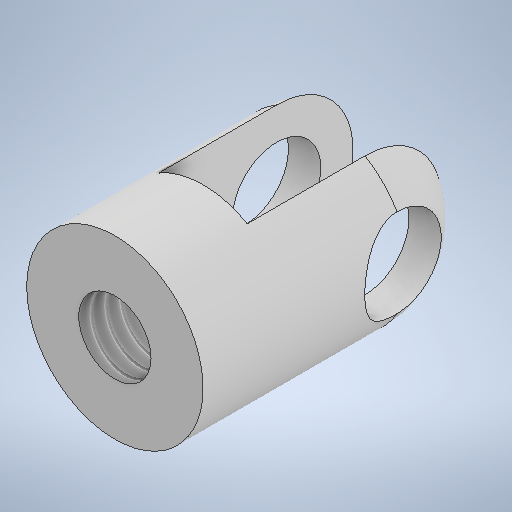
# Autodesk Inventor part: 19.1
Saved by Autodesk Inventor 2025.1 (Build 291241000, 241)
## iProperties
Created: 2024-09-13
Part Number: 19.1
Material: Generisch
Document SubType Name: Modeling
Designer: ffogue
Density: 1 g/cm^3
Appearance: Vorgabe
Author: ffogue
Autodesk Inventor part; units mm, degrees
ref_plane "XZ Plane" through (0, 0, 0) normal (0, 1, 0) x (-1, 0, 0)
sketch "Sketch1" plane through (0, 0, 0) normal (0, 1, 0) x (-1, 0, 0)
  circle A0 centre (0, 0) radius 3
  dimension "d0" = 6
  constraints: 1 centre point, 1 coincident
  measures "d0" diameter of A0
extrude "Extrusion1" add sketch "Sketch1" along normal blind 10
fillet "Fillet1" radius 3 1 edges at (3, 10, 0)
ref_plane "Work Plane2" through (0, 0, 3) normal (0, 0, 1) x (1, 0, 0)
ref_plane "Work Plane3" through (3, 0, 0) normal (1, 0, 0) x (0, 1, 0)
sketch "Sketch6" plane through (3, 0, 0) normal (1, 0, 0) x (0, 1, 0)
  circle A0 centre (7, 0) radius 1.5
  arc A1 (7, -3) -> (7, 3) centre (7, 0) ccw projected
  point P0 (0, 0)
  dimension "d21" = 3
  constraints: 1 centre point, 1 coincident
  measures "d21" diameter of A0
extrude "Extrusion4" cut sketch "Sketch6" against normal blind 6
sketch "Sketch5" plane through (0, 0, 3) normal (0, 0, 1) x (1, 0, 0)
  line L0 (3, 0) -> (-3, 0) projected
  line L1 (-1.5, 9.5981) -> (-1.5, 3)
  line L2 (-1.5, 3) -> (1.5, 3)
  line L3 (1.5, 3) -> (1.5, 9.5981)
  arc A0 (2.5981, 8.5) -> (-2.5981, 8.5) centre (0, 7) ccw projected
  line L4 (0, 3) -> (0, 10) construction
  line L5 (2.5981, 7) -> (-2.5981, 7) projected
  arc A1 (1.4921, 9.6026) -> (-1.5, 9.5981) centre (0, 7) ccw
  point P0 (0, 0)
  point P1 (3, 10)
  point P2 (-3, 10)
  point P3 (0, 9.7895)
  point P4 (0, 10)
  point P5 (0, 0)
  dimension "d16" = 3
  dimension "d25" = 7
  dimension "d26" = 1.5
  constraints: 8 end point, 8 point on circle, 3 midpoint, 2 vertical alignment, 1 centre point, 1 concentric, 1 horizontal alignment, 1 perpendicular, 1 other
  measures "d16" distance of L1.end L2.end
  measures "d25" distance from line of L2 point (0, 10)
  measures "d26" distance from line of point (0, 0) L1
extrude "Extrusion3" cut sketch "Sketch5" against normal blind 6
sketch "Sketch7" plane through (0, 0, 0) normal (0, -1, 0) x (1, 0, 0)
  circle A0 centre (0, 0) radius 3 projected
  constraints: 1 coincident
hole "Hole2" at (0, 0, 0) direction (0, 1, 0) diameter 2.459 depth 3 thread size "M3x0.5" class "6H" standard "ISO Metric profile"
body "Solid1"
